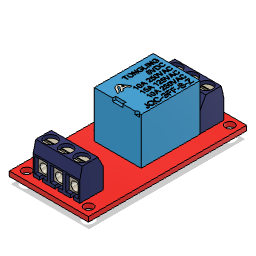
5V One Channel Relay (Autodesk Fusion 360 design; units mm, degrees)
Autodesk Fusion 360 part; units mm, degrees
note: some values were not read from the file. Chosen so that the rebuilt part matches the saved one: which bodies a step acts on; that a step has no effect.
sketch "Sketch1" plane through (0, 0, 0) normal (0, 1, 0) x (1, 0, 0)
  line L0 (0, 0) -> (25.5, 0)
  line L1 (25.5, 0) -> (25.5, 51)
  line L2 (25.5, 51) -> (0, 51)
  line L3 (0, 51) -> (0, 0)
  line L4 (2.75, 51) -> (2.75, 0) construction
  circle A0 centre (2.75, 48.325) radius 1.475
  circle A1 centre (2.75, 2.825) radius 1.475
  line L5 (12.75, 51) -> (12.75, 0) construction
  circle A2 centre (22.75, 48.325) radius 1.475
  circle A3 centre (22.75, 2.825) radius 1.475
  dimension "d1" = 25.5
  dimension "d2" = 51
  dimension "d3" = 2.95
  dimension "d4" = 1.275
  dimension "d5" = 1.2
  dimension "d7" = 2.75
  dimension "d270" = 45.5
  dimension "d271" = 20
  constraint horizontal L0
  constraint vertical L1
  constraint horizontal L2
  constraint vertical L3
  constraint coincident L0.start L3.end
  constraint coincident L2 L4.start
  constraint coincident L0 L4.end
  constraint perpendicular L0 L4
  constraint coincident L4 A0.centre
  constraint coincident L4 A1.centre
  constraint equal A0 A1
  constraint midpoint L2 L5.start
  constraint midpoint L0 L5.end
  constraint symmetric A0 L5 A2
  constraint symmetric A1 L5 A3
  measures "d1" distance of L0.start L0.end
  measures "d2" distance of L0.start L2.end
  measures "d3" diameter of A0
  measures "d4" distance of L3 A0
  measures "d5" distance of L2 A0
  measures "d7" distance of L3 L4
  measures "d270" distance of A0.centre A1.centre
  measures "d271" distance of A1.centre A3.centre
extrude "Extrude1" add sketch "Sketch1" along normal blind 1.55 makes body 1
sketch "Sketch2" plane through (0, 1.55, 0) normal (0, 1, 0) x (-1, 0, 0)
  circle A0 centre (-2.75, -2.825) radius 1.475
  circle A1 centre (-22.75, -2.825) radius 1.475
  circle A2 centre (-22.75, -48.325) radius 1.475
  circle A3 centre (-2.75, -48.325) radius 1.475
  line L0 (0, -51) -> (0, 0)
  line L1 (0, 0) -> (-25.5, 0)
  line L2 (-25.5, 0) -> (-25.5, -51)
  line L3 (-25.5, -51) -> (0, -51)
  line L4 (-5.4, -41) -> (-20.5, -41)
  line L5 (-20.5, -41) -> (-20.5, -22)
  line L6 (-20.5, -22) -> (-5.4, -22)
  line L7 (-5.4, -22) -> (-5.4, -41)
  dimension "d14" = 15.1
  dimension "d15" = 19
  dimension "d16" = 10
  dimension "d17" = 5
  dimension "d18" = 5.4
  dimension "d19" = 22
  constraint horizontal L4
  constraint vertical L5
  constraint horizontal L6
  constraint vertical L7
  measures "d14" distance of L4.start L4.end
  measures "d15" distance of L4.start L6.end
  measures "d16" distance of L3 L4
  measures "d17" distance of L2 L5
  measures "d18" distance of L0 L7
  measures "d19" distance of L1 L6
extrude "Extrude2" add sketch "Sketch2" along normal blind 15 separate body contours L4 L5 L6 L7 makes body 2
sketch "Sketch3" plane through (0, 16.55, 0) normal (0, 1, 0) x (-1, 0, 0)
  line L0 (-5.4, -22) -> (-20.5, -22)
  line L1 (-20.5, -22) -> (-20.5, -41)
  line L2 (-20.5, -41) -> (-5.4, -41)
  line L3 (-5.4, -41) -> (-5.4, -22)
  circle A0 centre (-19.25, -21.75) radius 0.75
  line L4 (-14.6, -23) -> (-11.3, -23)
  line L5 (-11.3, -23) -> (-11.3, -21)
  line L6 (-11.3, -21) -> (-14.6, -21)
  line L7 (-14.6, -21) -> (-14.6, -23)
  line L8 (-14.6, -23) -> (-11.3, -21) construction
  line L9 (-11.3, -23) -> (-14.6, -21) construction
  point P0 (-12.95, -22)
  dimension "d22" = 1.5
  dimension "d23" = 0.5
  dimension "d24" = 0.5
  dimension "d25" = 1
  dimension "d26" = 3.3
  constraint horizontal L4
  constraint perpendicular L4 L5
  constraint parallel L4 L6
  constraint parallel L5 L7
  constraint coincident L8 P0
  constraint coincident L9 P0
  constraint midpoint L0 P0
  measures "d22" diameter of A0
  measures "d23" distance of L0 A0
  measures "d24" distance of L1 A0
  measures "d25" distance of L0 L4
  measures "d26" distance of L5.end L6.end
extrude "Extrude3" cut sketch "Sketch3" against normal blind 1 contours L0 L4 L5 L7 | L0 L5 L6 L7 | L0 A0 | L0 A0 bodies 2
sketch "Sketch4" plane through (0, 16.55, 0) normal (0, 1, 0) x (-1, 0, 0)
  line L0 (-11.3, -22) -> (-11.3, -23)
  line L1 (-11.3, -23) -> (-14.6, -23)
  line L2 (-14.6, -23) -> (-14.6, -22)
  line L3 (-14.6, -22) -> (-18.5429, -22)
  line L4 (-20.5, -22) -> (-20.5, -41)
  line L5 (-20.5, -41) -> (-5.4, -41)
  line L6 (-5.4, -41) -> (-5.4, -22)
  line L7 (-5.4, -22) -> (-11.3, -22)
  arc A0 (-19.9571, -22) -> (-18.5429, -22) centre (-19.25, -21.75) ccw
  line L8 (-19.9571, -22) -> (-20.5, -22)
sketch "Sketch5" plane through (0, 1.55, 0) normal (0, 1, 0) x (-1, 0, 0)
  circle A0 centre (-2.75, -2.825) radius 1.475
  circle A1 centre (-22.75, -2.825) radius 1.475
  circle A2 centre (-22.75, -48.325) radius 1.475
  circle A3 centre (-2.75, -48.325) radius 1.475
  line L0 (0, -51) -> (0, 0)
  line L1 (0, 0) -> (-25.5, 0)
  line L2 (-25.5, 0) -> (-25.5, -51)
  line L3 (-25.5, -51) -> (0, -51)
  line L4 (-12.88, -3.54) -> (-20.5, -3.54)
  line L5 (-20.5, -3.54) -> (-20.5, -1)
  line L6 (-20.5, -1) -> (-12.88, -1)
  line L7 (-12.88, -1) -> (-12.88, -3.54)
  line L8 (-15.42, -3.54) -> (-15.42, -1) construction
  line L9 (-17.96, -3.54) -> (-17.96, -1) construction
  line L10 (-14.912, -3.54) -> (-15.42, -3.032)
  line L11 (-16.69, -3.54) -> (-16.69, -1) construction
  line L12 (-12.88, -2.27) -> (-16.69, -2.27) construction
  line L13 (-14.15, -3.54) -> (-14.15, -1) construction
  line L14 (-12.88, -3.032) -> (-13.388, -3.54)
  line L15 (-15.928, -3.54) -> (-15.42, -3.032)
  line L16 (-12.88, -1.508) -> (-13.388, -1)
  line L17 (-14.912, -1) -> (-15.42, -1.508)
  line L18 (-15.928, -1) -> (-15.42, -1.508)
  line L19 (-20.5, -3.032) -> (-19.992, -3.54)
  line L20 (-20.5, -1.508) -> (-19.992, -1)
  line L21 (-18.468, -1) -> (-17.96, -1.508)
  line L22 (-18.468, -3.54) -> (-17.96, -3.032)
  line L23 (-17.452, -3.54) -> (-17.96, -3.032)
  line L24 (-17.452, -1) -> (-17.96, -1.508)
  dimension "d29" = 7.62
  dimension "d30" = 2.54
  dimension "d31" = 5
  dimension "d32" = 1
  dimension "d33" = 2.54
  dimension "d34" = 2.54
  dimension "d35" = 45
  dimension "d36" = 0.508
  dimension "d37" = 1.27
  dimension "d38" = 45
  constraint horizontal L4
  constraint vertical L5
  constraint horizontal L6
  constraint vertical L7
  constraint coincident L4 L8.start
  constraint coincident L6 L8.end
  constraint perpendicular L6 L8
  constraint coincident L4 L9.start
  constraint coincident L6 L9.end
  constraint perpendicular L6 L9
  constraint coincident L4 L10.start
  constraint coincident L8 L10.end
  constraint midpoint L4 L11.start
  constraint midpoint L6 L11.end
  constraint midpoint L7 L12.start
  constraint midpoint L11 L12.end
  constraint coincident L4 L13.start
  constraint coincident L6 L13.end
  constraint perpendicular L6 L13
  constraint coincident L7 L14.start
  constraint coincident L4 L14.end
  constraint horizontal L10.end L14.start
  constraint symmetric L8 L10.start L15.start
  constraint symmetric L8 L10.end L15.end
  constraint symmetric L10.start L12 L17.start
  constraint symmetric L10.end L12 L17.end
  constraint symmetric L12 L14.start L16.start
  constraint symmetric L12 L14.end L16.end
  constraint symmetric L12 L15.start L18.start
  constraint symmetric L12 L10.end L17.end
  constraint symmetric L10.start L11 L22.start
  constraint symmetric L10.end L11 L22.end
  constraint symmetric L11 L14.start L19.start
  constraint symmetric L11 L14.end L19.end
  constraint symmetric L11 L15.start L23.start
  constraint symmetric L11 L10.end L22.end
  constraint symmetric L11 L16.start L20.start
  constraint symmetric L11 L16.end L20.end
  constraint symmetric L11 L17.start L21.start
  constraint symmetric L11 L17.end L21.end
  constraint symmetric L11 L18.start L24.start
  measures "d29" distance of L4.start L4.end
  measures "d30" distance of L4.start L6.end
  measures "d31" distance of L2 L5
  measures "d32" distance of L1 L6
  measures "d33" distance of L8 L9
  measures "d34" distance of L7 L8
  measures "d35" angle of L8 L10
  measures "d36" distance of L8.start L10.end
  measures "d37" distance of L7 L13
  measures "d38" angle of L7 L14
ref_plane "WorkPlane1" through (12.75, 0.775, 5) normal (0, 0, 1) x (1, 0, 0)
sketch "Sketch12" plane through (5.4, 0, 0) normal (-1, 0, 0) x (0, 0, 1)
  line L0 (-41, 1.55) -> (-22, 1.55)
  line L1 (-22, 1.55) -> (-22, 16.55)
  line L2 (-22, 16.55) -> (-41, 16.55)
  line L3 (-41, 16.55) -> (-41, 1.55)
  line L4 (-48.7, 1.55) -> (-41.1, 1.55)
  line L5 (-41.1, 1.55) -> (-41.1, 8.05)
  line L6 (-48.7, 8.05) -> (-48.7, 1.55)
  line L7 (-51, 1.55) -> (0, 1.55)
  line L8 (-47.9, 11.55) -> (-42.9, 11.55)
  line L9 (-47.9, 11.55) -> (-48.7, 8.05)
  line L10 (-42.9, 11.55) -> (-41.1, 8.05)
  line L11 (-48.7, 8.05) -> (-41.1, 8.05) construction
  dimension "d83" = 7.6
  dimension "d84" = 6.5
  dimension "d85" = 0.1
  dimension "d86" = 5
  dimension "d89" = 1.8
  dimension "d90" = 3.5
  constraint horizontal L4
  constraint vertical L5
  constraint vertical L6
  constraint collinear L4 L7
  constraint horizontal L8
  constraint horizontal L5.end L6.start
  measures "d83" distance of L4.start L4.end
  measures "d84" distance of L4.start L6.start
  measures "d85" distance of L3 L5
  measures "d86" distance of L8.start L8.end
  measures "d89" horizontal distance of L5.end L8.end
  measures "d90" distance of L6.start L8
extrude "Extrude8" add sketch "Sketch12" against normal blind 15 separate body contours L4 L5 L6 L7 L8 L9 L10 makes body 3
sketch "Sketch13" plane through (0, 0, -48.7) normal (0, 0, -1) x (-1, 0, 0)
  line L0 (-5.4, 1.55) -> (-5.4, 8.05)
  line L1 (-5.4, 8.05) -> (-20.4, 8.05)
  line L2 (-20.4, 8.05) -> (-20.4, 1.55)
  line L3 (-20.4, 1.55) -> (-5.4, 1.55)
  line L4 (-19.9, 7.55) -> (-15.9, 7.55)
  line L5 (-15.9, 7.55) -> (-15.9, 2.55)
  line L6 (-15.9, 2.55) -> (-19.9, 2.55)
  line L7 (-19.9, 2.55) -> (-19.9, 7.55)
  dimension "d93" = 4
  dimension "d94" = 5
  dimension "d95" = 0.5
  dimension "d97" = 1
  constraint horizontal L4
  constraint vertical L5
  constraint horizontal L6
  constraint vertical L7
  measures "d93" distance of L4.start L4.end
  measures "d94" distance of L4.start L6.end
  measures "d95" distance of L2 L7
  measures "d97" distance of L3 L6
extrude "Extrude9" cut sketch "Sketch13" against normal blind 5.8 contours L4 L5 L6 L7 bodies 3
pattern_linear "R-Pattern2" count 3 spacing 5 along (-1, 0, 0) of "Extrude9"
sketch "Sketch14" plane through (0, 11.55, 0) normal (0, 1, 0) x (-1, 0, 0)
  line L0 (-5.4, -47.9) -> (-5.4, -42.9)
  line L1 (-5.4, -42.9) -> (-20.4, -42.9)
  line L2 (-20.4, -42.9) -> (-20.4, -47.9)
  line L3 (-20.4, -47.9) -> (-5.4, -47.9)
  line L4 (-20.4, -45.6) -> (-5.4, -45.6) construction
  line L5 (-5.4, -41.1) -> (-20.4, -41.1) construction
  circle A0 centre (-17.9, -45.6) radius 2
  dimension "d104" = 4.5
  dimension "d105" = 4
  dimension "d106" = 0.5
  constraint coincident L2 L4.start
  constraint coincident L0 L4.end
  constraint perpendicular L0 L4
  constraint coincident L4 A0.centre
  measures "d104" distance of L4 L5
  measures "d105" diameter of A0
  measures "d106" distance of L2 A0
extrude "Extrude10" cut sketch "Sketch14" against normal up to surface (4 mm away) contours A0 bodies 3
pattern_linear "R-Pattern3" count 3 spacing 5 along (-1, 0, 0) of "Extrude10"
sketch "Sketch15" plane through (0, 2.55, 0) normal (0, 1, 0) x (-1, 0, 0)
  line L0 (-19.9, -48.7) -> (-15.9, -48.7)
  line L1 (-15.9, -48.7) -> (-15.9, -42.9)
  line L2 (-15.9, -42.9) -> (-19.9, -42.9)
  line L3 (-19.9, -42.9) -> (-19.9, -48.7)
  line L4 (-5.4, -41.1) -> (-20.4, -41.1)
  line L5 (-17.4, -45.6) -> (-17.4, -48.7)
  line L6 (-18.4, -48.7) -> (-18.4, -45.6)
  arc A0 (-17.4, -45.6) -> (-18.4, -45.6) centre (-17.9, -45.6) ccw
  line L7 (-17.4, -48.7) -> (-18.4, -48.7)
  dimension "d113" = 1
  dimension "d114" = 4.5
  dimension "d115" = 2
  constraint coincident L0 L5.end
  constraint perpendicular L0 L5
  constraint coincident L0 L6.start
  constraint vertical L6
  constraint tangent L5 A0
  constraint tangent L6 A0
  measures "d113" diameter of A0
  measures "d114" distance of A0.centre L4
  measures "d115" distance of L3 A0.centre
extrude "Extrude11" cut sketch "Sketch15" against normal up to surface (1 mm away) contours L0 L5 L6 A0 L7 bodies 3
pattern_linear "R-Pattern4" count 3 spacing 5 along (-1, 0, 0) of "Extrude11"
sketch "Sketch16" plane through (0, 0, -42.9) normal (0, 0, -1) x (-1, 0, 0)
  line L0 (-19.9, 2.55) -> (-15.9, 2.55)
  line L1 (-15.9, 2.55) -> (-15.9, 7.55)
  line L2 (-15.9, 7.55) -> (-19.9, 7.55)
  line L3 (-19.9, 7.55) -> (-19.9, 2.55)
  line L4 (-17.9, 7.55) -> (-17.9, 2.55) construction
  circle A0 centre (-17.9, 4.45) radius 1.4
  line L5 (-18.4, 1.55) -> (-20.4, 1.55)
  dimension "d122" = 2.8
  dimension "d123" = 2.9
  constraint midpoint L2 L4.start
  constraint midpoint L0 L4.end
  constraint coincident L4 A0.centre
  measures "d122" diameter of A0
  measures "d123" distance of A0.centre L5
extrude "Extrude12" add sketch "Sketch16" along normal blind 4.7 separate body makes body 4
ref_plane "WorkPlane3" through (12.9, -2.2, -44.9) normal (0, -1, 0) x (0, 0, -1)
sketch "Sketch17" plane through (13.4, -2.2, -27.4) normal (0, -1, 0) x (1, 0, 0)
  circle A0 centre (4.5, -18.2) radius 0.5
  arc A1 (5, -18.2) -> (4, -18.2) centre (4.5, -18.2) ccw
  dimension "d127" = 1
  constraint concentric A0 A1
  measures "d127" diameter of A0
extrude "Extrude13" add sketch "Sketch17" against normal up to surface (4.75 mm away) separate body makes body 5
combine "Combine3" operation add target body 4 tool bodies 5
sketch "Sketch18" plane through (0, 7.55, 0) normal (0, 1, 0) x (-1, 0, 0)
  line L0 (-15.9, -42.9) -> (-19.9, -42.9)
  line L1 (-19.9, -42.9) -> (-19.9, -47.6)
  line L2 (-19.9, -47.6) -> (-15.9, -47.6)
  line L3 (-15.9, -47.6) -> (-15.9, -42.9)
  circle A0 centre (-17.9, -45.6) radius 0.84
  circle A1 centre (-17.9, -45.6) radius 2
  dimension "d130" = 1.68
  constraint concentric A0 A1
  measures "d130" diameter of A0
extrude "Extrude14" cut sketch "Sketch18" along normal up to surface contours A0 end surface at (16.5017, 4.3802, -46.0333) on bodies 4 bodies 4
ref_plane "WorkPlane4" through (12.9, 8.55, -45.4) normal (0, 1, 0) x (0, 0, 1)
sketch "Sketch21" plane through (13.4, 8.55, -27.9) normal (0, 1, 0) x (1, 0, 0)
  circle A0 centre (4.5, 17.7) radius 0.84
extrude "Extrude15" add sketch "Sketch21" against normal blind 3 separate body makes body 6
sketch "Sketch22" plane through (0, 8.55, 0) normal (0, 1, 0) x (-1, 0, 0)
  circle A0 centre (-17.9, -45.6) radius 0.84
  circle A1 centre (-17.9, -45.6) radius 2
extrude "Extrude16" add sketch "Sketch22" along normal blind 2 separate body contours A0 | A1 makes body 7
combine "Combine4" operation add target body 6 tool bodies 7
sketch "Sketch23" plane through (0, 10.55, 0) normal (0, 1, 0) x (-1, 0, 0)
  circle A0 centre (-17.9, -45.6) radius 2
  line L0 (-17.9, -45.6) -> (-19.9, -45.6) construction
  line L1 (-19.8645, -45.975) -> (-15.9355, -45.975)
  line L2 (-15.9355, -45.225) -> (-19.8645, -45.225)
  arc A1 (-15.9355, -45.975) -> (-15.9355, -45.225) centre (-17.9, -45.6) ccw
  arc A2 (-19.8645, -45.225) -> (-19.8645, -45.975) centre (-17.9, -45.6) ccw
  dimension "d138" = 0.75
  dimension "d139" = 0.375
  dimension "d140" = 2
  dimension "d141" = 2
  constraint coincident A0.centre L0.start
  constraint coincident A0 L0.end
  constraint horizontal L0
  constraint horizontal L1
  constraint horizontal L2
  constraint coincident A0 L2.start
  constraint coincident A0 L1.start
  constraint concentric A1 A2
  measures "d138" distance of L1 L2
  measures "d139" distance of L0 L2
  measures "d140" radius of A1
  measures "d141" radius of A2
extrude "Extrude17" cut sketch "Sketch23" against normal blind 0.3 contours A0 L1 L2 A1 A2 bodies 6
pattern_linear "R-Pattern5" count 3 spacing 5 along (-1, 0, 0) of bodies 4 6 makes body 8 at (13.8675, 5.4619, -45.3721) makes body 9 at (8.8675, 5.4619, -45.3721) makes body 10 at (11.0287, 9.2167, -46.3059) makes body 11 at (6.0287, 9.2167, -46.3059)
combine "Combine5" operation cut target body 1 tool bodies 4 8 9 keep tools
combine "Combine6" operation add target body 4 tool bodies 6
combine "Combine7" operation add target body 8 tool bodies 10
combine "Combine8" operation add target body 9 tool bodies 11
sketch "Sketch24" plane through (0, 0, 0) normal (0, -1, 0) x (1, 0, 0)
  circle A0 centre (7.9, -45.6) radius 0.5
  circle A1 centre (12.9, -45.6) radius 0.5
  circle A2 centre (17.9, -45.6) radius 0.5
  circle A3 centre (2.75, -2.825) radius 1.475
  circle A4 centre (22.75, -2.825) radius 1.475
  circle A5 centre (22.75, -48.325) radius 1.475
  circle A6 centre (2.75, -48.325) radius 1.475
  line L0 (0, 0) -> (0, -51)
  line L1 (0, -51) -> (25.5, -51)
  line L2 (25.5, -51) -> (25.5, 0)
  line L3 (25.5, 0) -> (0, 0)
  circle A7 centre (18.95, -25.4) radius 0.65
  line L4 (6.95, -37.6) -> (18.95, -37.6) construction
  circle A8 centre (6.95, -37.6) radius 0.65
  circle A9 centre (18.95, -37.6) radius 0.65
  circle A10 centre (6.95, -25.4) radius 0.65
  line L5 (6.95, -25.4) -> (18.95, -25.4) construction
  line L6 (20.5, -22) -> (5.4, -22) construction
  line L7 (5.4, -22) -> (5.4, -41) construction
  line L8 (5.4, -41) -> (20.5, -41) construction
  line L9 (20.5, -41) -> (20.5, -22) construction
  line L10 (12.95, -41) -> (12.95, -22) construction
  circle A11 centre (12.95, -23.4) radius 0.65
  dimension "d148" = 1.3
  dimension "d151" = 12
  dimension "d152" = 12
  dimension "d153" = 12.2
  dimension "d157" = 3.4
  dimension "d158" = 2
  constraint horizontal L4
  constraint coincident L4.start A8.centre
  constraint coincident L4.end A9.centre
  constraint coincident A10.centre L5.start
  constraint coincident A7.centre L5.end
  constraint equal A9 A10
  constraint equal A7 A10
  constraint midpoint L8 L10.start
  constraint midpoint L6 L10.end
  constraint symmetric L4.start L4.end L10
  constraint symmetric A7.centre A10.centre L10
  constraint coincident L10 A11.centre
  constraint equal A7 A11
  measures "d148" diameter of A7
  measures "d151" distance of A10.centre A7.centre
  measures "d152" distance of L4.start L4.end
  measures "d153" distance of A7.centre L4.end
  measures "d157" distance of L4.end L8
  measures "d158" distance of L5 A11.centre
extrude "Extrude19" add sketch "Sketch24" along normal blind 2 and the other way up to surface (1.55 mm away) separate body contours A7 | A8 | A9 | A10 | A11 makes body 12 at (18.3201, -1.3333, -25.5604) makes body 13 at (19.5046, -1.3333, -37.2611) makes body 14 at (13.5992, -1.3333, -23.4324) makes body 15 at (7.5046, -1.3333, -37.9389) makes body 16 at (7.549, -1.3333, -25.1475)
sketch "Sketch26" plane through (0, 16.55, 0) normal (0, 1, 0) x (-1, 0, 0)
  line L0 (-11.3, -22) -> (-11.3, -23)
  line L1 (-11.3, -23) -> (-14.6, -23)
  line L2 (-14.6, -23) -> (-14.6, -22)
  line L3 (-14.6, -22) -> (-18.5429, -22)
  line L4 (-20.5, -22) -> (-20.5, -41)
  line L5 (-20.5, -41) -> (-5.4, -41)
  line L6 (-5.4, -41) -> (-5.4, -22)
  line L7 (-5.4, -22) -> (-11.3, -22)
  line L8 (-9.8102, -26.6279) -> (-9.8687, -27.3586)
  line L9 (-9.8687, -27.3586) -> (-9.1687, -26.9586)
  line L10 (-9.1687, -26.9586) -> (-9.8102, -26.6279)
  line L11 (-10.3687, -26.2086) -> (-10.4687, -27.4586)
  line L12 (-11.0687, -27.9086) -> (-11.0687, -28.3586)
  line L13 (-11.0187, -28.4086) -> (-10.7687, -28.4086)
  line L14 (-10.554, -24.1615) -> (-10.7674, -24.1615)
  line L15 (-10.8174, -24.2115) -> (-10.8174, -24.5086)
  spline S0 degree 5 poles (-10.554, -24.1615) (-10.4508, -24.2403) (-10.247, -24.3884) (-9.9485, -24.582) (-9.5673, -24.7909) (-9.1325, -25.0111) (-8.7616, -25.2377) (-8.4801, -25.5077) (-8.324, -25.8344) (-8.3206, -26.1829) (-8.3742, -26.4864) (-8.4086, -26.7014) (-8.4512, -26.854) (-8.7491, -27.0949) (-9.2801, -27.4323) (-9.9251, -27.8223) (-10.3857, -28.1118) (-10.627, -28.2826) (-10.7309, -28.3708) (-10.7687, -28.4086) knots 0 0 0 0 0 0 0.066667 0.133333 0.2 0.266667 0.333333 0.4 0.466667 0.533333 0.6 0.666667 0.733333 0.8 0.866667 0.933333 1 1 1 1 1 1
  line L16 (-11.1393, -23.7145) -> (-9.9687, -24.6086)
  line L17 (-8.6581, -25.225) -> (-8.2199, -26.0488)
  line L18 (-8.3375, -26.5355) -> (-8.5387, -26.9881)
  line L19 (-10.5687, -28.2086) -> (-10.9687, -28.6086)
  spline S1 degree 5 poles (-10.8174, -24.5086) (-10.8147, -24.53) (-10.8056, -24.5728) (-10.781, -24.6373) (-10.7261, -24.7236) (-10.6204, -24.8321) (-10.4784, -24.9415) (-10.303, -25.0521) (-10.1011, -25.1647) (-9.8831, -25.2801) (-9.6616, -25.3993) (-9.4498, -25.5235) (-9.2598, -25.6536) (-9.1017, -25.7904) (-8.981, -25.9341) (-8.9001, -26.0848) (-8.8676, -26.2109) (-8.8612, -26.3086) (-8.8649, -26.375) (-8.8687, -26.4086) knots 0 0 0 0 0 0 0.066667 0.133333 0.2 0.266667 0.333333 0.4 0.466667 0.533333 0.6 0.666667 0.733333 0.8 0.866667 0.933333 1 1 1 1 1 1
  spline S2 degree 5 poles (-8.8687, -26.4086) (-8.9139, -26.3886) (-9.0038, -26.3482) (-9.1364, -26.2863) (-9.3091, -26.2009) (-9.5175, -26.0892) (-9.7178, -25.972) (-9.9092, -25.849) (-10.0914, -25.7197) (-10.2646, -25.5845) (-10.4295, -25.4437) (-10.5553, -25.3271) (-10.6465, -25.2374) (-10.7058, -25.1767) (-10.7352, -25.1461) knots 0 0 0 0 0 0 0.1 0.2 0.3 0.4 0.5 0.6 0.7 0.8 0.9 1 1 1 1 1 1
  spline S3 degree 5 poles (-10.7352, -25.1461) (-10.7552, -25.1414) (-10.7931, -25.1346) (-10.843, -25.1325) (-10.896, -25.146) (-10.9398, -25.1897) (-10.9639, -25.2578) (-10.9739, -25.3454) (-10.9822, -25.441) (-10.9909, -25.5382) (-10.9957, -25.6332) (-10.9886, -25.7248) (-10.9609, -25.8128) (-10.9061, -25.8977) (-10.821, -25.9796) (-10.7042, -26.0587) (-10.5856, -26.1199) (-10.4825, -26.1647) (-10.4077, -26.194) (-10.3687, -26.2086) knots 0 0 0 0 0 0 0.066667 0.133333 0.2 0.266667 0.333333 0.4 0.466667 0.533333 0.6 0.666667 0.733333 0.8 0.866667 0.933333 1 1 1 1 1 1
  line L20 (-10.9465, -25.1504) -> (-10.9909, -25.4668)
  arc A0 (-10.7674, -24.1615) -> (-10.8174, -24.2115) centre (-10.7674, -24.2115) ccw
  arc A1 (-11.0687, -28.3586) -> (-11.0187, -28.4086) centre (-11.0187, -28.3586) ccw
  spline S4 degree 5 poles (-10.4687, -27.4586) (-10.4899, -27.4686) (-10.5326, -27.4896) (-10.5976, -27.524) (-10.6864, -27.5757) (-10.8027, -27.655) (-10.9024, -27.7376) (-10.983, -27.8158) (-11.0396, -27.8762) (-11.0687, -27.9086) knots 0 0 0 0 0 0 0.2 0.4 0.6 0.8 1 1 1 1 1 1
  line L21 (-10.9953, -27.8269) -> (-11.1421, -27.9902)
  line L22 (-8.55, -29.0893) -> (-8.55, -40) construction
  line L23 (-10.75, -40) -> (-10.75, -17.7062) construction
  line L24 (-5.4, -40) -> (-20.5, -40) construction
  line L25 (-12.95, -27.9754) -> (-12.95, -40) construction
  line L26 (-15.15, -27.9773) -> (-15.15, -40) construction
  line L27 (-17.35, -27.9531) -> (-17.35, -40) construction
  line L28 (-19.85, -24.6083) -> (-19.85, -40) construction
  arc A2 (-19.9571, -22) -> (-18.5429, -22) centre (-19.25, -21.75) ccw
  line L29 (-19.9571, -22) -> (-20.5, -22)
  point P0 (-8.439, -25.6369)
  point P1 (-8.4381, -26.7618)
  point P2 (-10.3687, -25.0086)
  point P3 (-9.2409, -25.6763)
  point P4 (-9.9201, -25.8385)
  point P5 (-10.9687, -25.3086)
  point P6 (-10.9718, -25.7684)
  dimension "d163" = 0.05
  dimension "d164" = 0.05
  dimension "d167" = 2.2
  dimension "d169" = 2.2
  dimension "d170" = 3.15
  dimension "d171" = 2.2
  dimension "d172" = 2.2
  dimension "d173" = 2.5
  dimension "d280" = 1
  constraint parallel L8 L11
  constraint vertical L12
  constraint perpendicular L12 L13
  constraint horizontal L14
  constraint perpendicular L14 L15
  constraint midpoint L14.start L16
  constraint midpoint P0 L17
  constraint midpoint P1 L18
  constraint midpoint L13.end L19
  constraint midpoint P5 L20
  constraint tangent L14 A0
  constraint tangent L15 A0
  constraint tangent L12 A1
  constraint tangent L13 A1
  constraint midpoint L12.start L21
  constraint vertical L22
  constraint perpendicular L5 L23
  constraint coincident L6 L24.start
  constraint coincident L4 L24.end
  constraint perpendicular L4 L24
  constraint coincident L22.end L24
  constraint coincident L23.start L24
  constraint midpoint L24 L25.end
  constraint vertical L25
  constraint coincident L24 L26.end
  constraint perpendicular L24 L26
  constraint coincident L24 L27.end
  constraint perpendicular L24 L27
  constraint coincident L24 L28.end
  constraint perpendicular L24 L28
  measures "d163" radius of A0
  measures "d164" radius of A1
  measures "d167" distance of L22 L23
  measures "d169" distance of L23 L25
  measures "d170" distance of L6 L22
  measures "d171" distance of L25 L26
  measures "d172" distance of L26 L27
  measures "d173" distance of L27 L28
  measures "d280" distance of L5.end L24.start
extrude "Extrude20" [no effect]
ref_plane "WorkPlane5" through (12.75, 1.75, -25.5) normal (0, 1, 0) x (1, 0, 0)
sketch "Sketch28" plane through (13, 1.75, -16.75) normal (0, 1, 0) x (1, 0, 0)
  line L0 (-8.5, 20.05) -> (-10.5, 20.05)
  line L1 (-10.5, 20.05) -> (-10.5, 16.05)
  line L2 (-10.5, 16.05) -> (-8.5, 16.05)
  line L3 (-8.5, 16.05) -> (-8.5, 20.05)
  line L4 (12.5, 34.25) -> (-13, 34.25)
  line L5 (7.5, 24.25) -> (-7.6, 24.25)
  line L6 (-13, 34.25) -> (-13, -16.75)
  dimension "d180" = 2
  dimension "d181" = 4
  dimension "d182" = 14.2
  dimension "d183" = 4.2
  dimension "d184" = 2.5
  constraint horizontal L0
  constraint vertical L1
  constraint horizontal L2
  constraint vertical L3
  measures "d180" distance of L0.start L0.end
  measures "d181" distance of L0.start L2.end
  measures "d182" distance of L0 L4
  measures "d183" distance of L0 L5
  measures "d184" distance of L1 L6
extrude "Extrude22" add sketch "Sketch28" along normal blind 2 separate body makes body 17
ref_plane "WorkPlane6" through (4, 2.75, -34.8) normal (-1, 0, 0) x (0, 0, 1)
sketch "Sketch29" plane through (4, 2.75, -17.3) normal (-1, 0, 0) x (0, 0, -1)
  line L0 (19.6, 1.2) -> (19.6, 0)
  line L1 (17.5, -1) -> (17.5, 1) construction
  line L2 (19.5, -1) -> (15.5, -1) construction
  line L3 (19.5, 1) -> (15.5, 1) construction
  line L4 (19.6, 0) -> (19.5, 0)
  line L5 (19.5, 1) -> (19.5, -1)
  line L6 (19.7, 1.2) -> (19.7, 0)
  line L7 (19.6, -0.1) -> (19.5, -0.1)
  arc A0 (19.6, -0.1) -> (19.7, 0) centre (19.6, 0) ccw
  line L8 (15.3, 1.2) -> (15.3, 0)
  arc A1 (15.3, 0) -> (15.4, -0.1) centre (15.4, 0) ccw
  line L9 (15.4, 0) -> (15.5, 0)
  line L10 (15.4, 1.2) -> (15.4, 0)
  line L11 (15.4, -0.1) -> (15.5, -0.1)
  line L12 (33.7, 1.2) -> (-17.3, 1.2)
  line L13 (19.7, 1.2) -> (19.6, 1.2)
  line L14 (15.4, 1.2) -> (15.3, 1.2)
  line L15 (15.5, -0.1) -> (15.5, 0)
  line L16 (19.5, -0.1) -> (19.5, 0)
  dimension "d188" = 0.1
  dimension "d190" = 0.1
  dimension "d191" = 0.1
  dimension "d192" = 0.1
  constraint vertical L0
  constraint vertical L1
  constraint midpoint L1.start L2
  constraint midpoint L1.end L3
  constraint perpendicular L0 L4
  constraint midpoint L4.end L5
  constraint parallel L0 L6
  constraint parallel L4 L7
  constraint tangent L6 A0
  constraint tangent L7 A0
  constraint symmetric L0.start L1 L10.start
  constraint symmetric L0.end L1 A1.centre
  constraint symmetric L1 L4.end L9.end
  constraint symmetric L1 L6.start L8.start
  constraint symmetric L1 L7.end L11.end
  constraint symmetric L1 L6.end L8.end
  constraint symmetric L1 L7.start A1.end
  constraint symmetric L1 A0 A1
  constraint coincident L6.start L12
  constraint coincident L0.start L12
  constraint coincident L5 L7.end
  measures "d188" distance of L0.end L4.end
  measures "d190" radius of A0
  measures "d191" distance of L0 L6
  measures "d192" distance of L4 L7
extrude "Extrude23" add sketch "Sketch29" along normal blind 1 separate body makes body 18 at (3.6667, 1.95, -37) makes body 19 at (3.6667, 1.95, -32.6)
sketch "Sketch30" plane through (0, 1.55, 0) normal (0, 1, 0) x (-1, 0, 0)
  circle A0 centre (-7.9, -45.6) radius 0.5
  circle A1 centre (-12.9, -45.6) radius 0.5
  circle A2 centre (-17.9, -45.6) radius 0.5
  circle A3 centre (-2.75, -2.825) radius 1.475
  circle A4 centre (-22.75, -2.825) radius 1.475
  circle A5 centre (-22.75, -48.325) radius 1.475
  circle A6 centre (-2.75, -48.325) radius 1.475
  line L0 (0, -51) -> (0, 0)
  line L1 (0, 0) -> (-25.5, 0)
  line L2 (-25.5, 0) -> (-25.5, -51)
  line L3 (-25.5, -51) -> (0, -51)
  line L4 (-4.5, -29.3) -> (-2.5, -29.3)
  line L5 (-2.5, -29.3) -> (-2.5, -28.3)
  line L6 (-2.5, -28.3) -> (-4.5, -28.3)
  line L7 (-4.5, -28.3) -> (-4.5, -29.3)
  line L8 (-4.5, -32.8) -> (-4.5, -36.8)
  line L9 (-2.5, -32.8) -> (-4.5, -32.8)
  dimension "d195" = 2
  dimension "d196" = 1
  dimension "d197" = 3.5
  constraint horizontal L4
  constraint vertical L5
  constraint horizontal L6
  constraint vertical L7
  constraint collinear L7 L8
  measures "d195" distance of L4.start L4.end
  measures "d196" distance of L4.start L6.end
  measures "d197" distance of L4 L9
extrude "Extrude24" add sketch "Sketch30" along normal blind 1 separate body contours L4 L5 L6 L7 makes body 20
sketch "Sketch31" plane through (0, 1.55, 0) normal (0, 1, 0) x (-1, 0, 0)
  circle A0 centre (-7.9, -45.6) radius 0.5
  circle A1 centre (-12.9, -45.6) radius 0.5
  circle A2 centre (-17.9, -45.6) radius 0.5
  circle A3 centre (-2.75, -2.825) radius 1.475
  circle A4 centre (-22.75, -2.825) radius 1.475
  circle A5 centre (-22.75, -48.325) radius 1.475
  circle A6 centre (-2.75, -48.325) radius 1.475
  line L0 (0, -51) -> (0, 0)
  line L1 (0, 0) -> (-25.5, 0)
  line L2 (-25.5, 0) -> (-25.5, -51)
  line L3 (-25.5, -51) -> (0, -51)
  line L4 (-3.75, -29.3) -> (-3.25, -29.3)
  line L5 (-3.25, -29.3) -> (-3.25, -29.8)
  line L6 (-3.25, -29.8) -> (-3.75, -29.8)
  line L7 (-3.75, -29.8) -> (-3.75, -29.3)
  line L8 (-3.5, -29.8) -> (-3.5, -28.3) construction
  line L9 (-2.5, -28.3) -> (-4.5, -28.3) construction
  line L10 (-4.5, -29.3) -> (-2.5, -29.3) construction
  line L11 (-4.5, -28.3) -> (-4, -28.3)
  line L12 (-4, -28.3) -> (-4, -27.8)
  line L13 (-4, -27.8) -> (-4.5, -27.8)
  line L14 (-4.5, -27.8) -> (-4.5, -28.3)
  line L15 (-3, -28.3) -> (-3, -27.8)
  line L16 (-2.5, -27.8) -> (-2.5, -28.3)
  line L17 (-3, -27.8) -> (-2.5, -27.8)
  line L18 (-2.5, -28.3) -> (-3, -28.3)
  point P0 (-2.5, -28.3)
  dimension "d200" = 0.5
  dimension "d201" = 0.5
  dimension "d202" = 0.5
  dimension "d203" = 0.5
  constraint horizontal L4
  constraint vertical L5
  constraint horizontal L6
  constraint vertical L7
  constraint midpoint L6 L8.start
  constraint perpendicular L6 L8
  constraint midpoint L8.end L9
  constraint collinear L4 L10
  constraint horizontal L11
  constraint vertical L12
  constraint horizontal L13
  constraint vertical L14
  constraint coincident L9.end L11.start
  constraint symmetric L8 L9.end P0
  constraint symmetric L8 L11.end L15.start
  constraint symmetric L8 L12.end L15.end
  constraint symmetric L8 L13.end L16.start
  measures "d200" distance of L5 L7
  measures "d201" distance of L4.start L6.end
  measures "d202" distance of L9.end L11.end
  measures "d203" distance of L9.end L13.end
extrude "Extrude25" add sketch "Sketch31" along normal blind 0.125 separate body contours L4 L5 L6 L7 | L11 L12 L13 L14 | L15 L16 L17 L18 makes body 21 at (3.4167, 1.55, -29.6333) makes body 22 at (2.8333, 1.55, -28.1333) makes body 23 at (4.3333, 1.55, -28.1333)
sketch "Sketch32" plane through (0, 1.55, 0) normal (0, 1, 0) x (-1, 0, 0)
  circle A0 centre (-7.9, -45.6) radius 0.5
  circle A1 centre (-12.9, -45.6) radius 0.5
  circle A2 centre (-17.9, -45.6) radius 0.5
  circle A3 centre (-2.75, -2.825) radius 1.475
  circle A4 centre (-22.75, -2.825) radius 1.475
  circle A5 centre (-22.75, -48.325) radius 1.475
  circle A6 centre (-2.75, -48.325) radius 1.475
  line L0 (0, -51) -> (0, 0)
  line L1 (0, 0) -> (-25.5, 0)
  line L2 (-25.5, 0) -> (-25.5, -51)
  line L3 (-25.5, -51) -> (0, -51)
  line L4 (-2.3, -26.5) -> (-3.3, -26.5)
  line L5 (-3.3, -26.5) -> (-3.3, -25)
  line L6 (-3.3, -25) -> (-2.3, -25)
  line L7 (-2.3, -25) -> (-2.3, -26.5)
  line L8 (-2.5, -29.3) -> (-2.5, -28.3)
  line L9 (-2.5, -28.3) -> (-4.5, -28.3)
  dimension "d206" = 1
  dimension "d207" = 1.5
  dimension "d208" = 0.2
  dimension "d209" = 1.8
  constraint horizontal L4
  constraint vertical L5
  constraint horizontal L6
  constraint vertical L7
  measures "d206" distance of L4.start L4.end
  measures "d207" distance of L4.start L6.end
  measures "d208" distance of L7 L8
  measures "d209" distance of L4 L9
extrude "Extrude26" add sketch "Sketch32" along normal blind 0.25 separate body contours L4 L5 L6 L7 makes body 24
sketch "Sketch33" plane through (2.3, 0, 0) normal (-1, 0, 0) x (0, 0, 1)
  line L0 (-26.5, 1.55) -> (-25, 1.55)
  line L1 (-25, 1.55) -> (-25, 1.8)
  line L2 (-25, 1.8) -> (-26.5, 1.8)
  line L3 (-26.5, 1.8) -> (-26.5, 1.55)
  line L4 (-25, 1.55) -> (-25, 1.6)
  line L5 (-25, 1.55) -> (-24.95, 1.55)
  arc A0 (-24.95, 1.55) -> (-25, 1.6) centre (-25, 1.55) ccw
  line L6 (-25.75, 1.8) -> (-25.75, 1.55) construction
  line L7 (-26.5, 1.55) -> (-26.5, 1.6)
  arc A1 (-26.5, 1.6) -> (-26.55, 1.55) centre (-26.5, 1.55) ccw
  line L8 (-26.5, 1.55) -> (-26.55, 1.55)
  dimension "d212" = 0.1
  constraint coincident L0.end L1.start
  constraint coincident L1 L4.end
  constraint perpendicular L0 L4
  constraint perpendicular L4 L5
  constraint midpoint L2 L6.start
  constraint midpoint L0 L6.end
  constraint symmetric L0.end L6 L0.start
  constraint symmetric L4.end L6 L7.end
  constraint symmetric L5.end L6 A1.end
  constraint symmetric A0 L6 A1
  measures "d212" diameter of A0
extrude "Extrude27" add sketch "Sketch33" against normal up to surface (1 mm away) separate body contours L3 L7 A1 L8 | L1 L4 L5 A0 makes body 25 at (2.9667, 1.5999, -24.9976) makes body 26 at (2.9667, 1.5845, -26.5362)
sketch "Sketch34" plane through (0, 1.8, 0) normal (0, 1, 0) x (-1, 0, 0)
  line L0 (-2.3, -25) -> (-3.3, -25)
  line L1 (-3.3, -25) -> (-3.3, -26.5)
  line L2 (-3.3, -26.5) -> (-2.3, -26.5)
  line L3 (-2.3, -26.5) -> (-2.3, -25)
  line L4 (-3.0427, -25) -> (-3.0427, -26.5) construction
  constraint coincident L0 L4.start
  constraint coincident L2 L4.end
  constraint perpendicular L2 L4
extrude "Extrude28" [no effect]
ref_plane "WorkPlane7" through (12.75, 0.775, -25.5) normal (0, 0, -1) x (-1, 0, 0)
mirror "Mirror1" about plane through (12.75, 0.775, -25.5) normal (0, 0, -1) of bodies 3 makes body 27
mirror "Mirror2" about plane through (12.75, 0.775, -25.5) normal (0, 0, -1) of bodies 4 makes body 28
mirror "Mirror3" about plane through (12.75, 0.775, -25.5) normal (0, 0, -1) of bodies 8 makes body 29
mirror "Mirror4" about plane through (12.75, 0.775, -25.5) normal (0, 0, -1) of bodies 9 makes body 30
equation "d29 = ( 2.54 * 3 ) * 1 mm"
equation "d36 = ( 2.54 / 5 ) * 1 mm"
equation "d37 = ( 2.54 / 2 ) * 1 mm"
equation "d98 = -( 7.6 mm - 1.8 mm )"
equation "d130 = ( ( 3 / 5 ) * 2.8 ) * 1 mm"
equation "d139 = ( 0.75 / 2 ) * 1 mm"
named bodies: "Board", "Relay", "Termial Block", "NO", "COM", "NC", "Termial Block (1)", "NO (1)", "COM (1)", "NC (1)"
